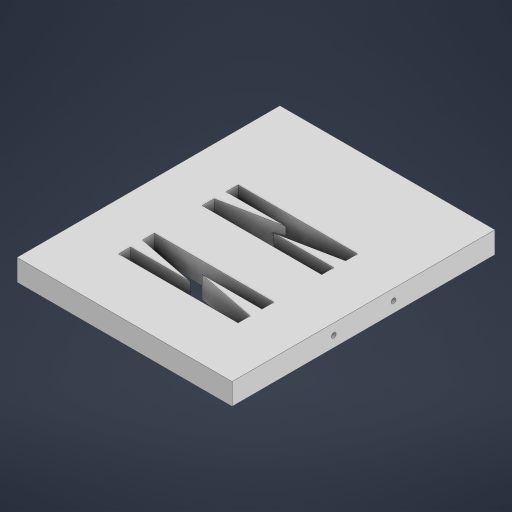
# Autodesk Inventor part: APM_001-3
Saved by Autodesk Inventor 2024 (Build 280153000, 153)
## iProperties
Created: 2023-05-12
Part Number: APM_001-3
Material: Genérico
Document SubType Name: Modeling
Designer: javie
Density: 1 g/cm^3
Appearance: Valor por defecto
Author: javie
Autodesk Inventor part; units mm, degrees
ref_plane "YZ Plane" through (0, 0, 0) normal (1, 0, 0) x (0, 1, 0)
ref_plane "XZ Plane" through (0, 0, 0) normal (0, 1, 0) x (-1, 0, 0)
ref_plane "XY Plane" through (0, 0, 0) normal (0, 0, 1) x (1, 0, 0)
sketch "Boceto1" plane through (0, 0, 0) normal (0, 1, 0) x (-1, 0, 0)
  line L0 (90, 220) -> (-90, 220)
  line L1 (-90, 220) -> (-90, 0)
  line L2 (-90, 0) -> (90, 0)
  line L3 (90, 0) -> (90, 220)
  line L4 (50, 175) -> (-50, 175)
  line L5 (-50, 175) -> (-50, 165)
  line L6 (50, 175) -> (50, 165)
  line L7 (50, 165) -> (0, 165)
  line L8 (50, 155) -> (50, 145)
  line L9 (50, 145) -> (-50, 145)
  line L10 (-50, 145) -> (-50, 155)
  line L11 (-50, 155) -> (0, 155)
  line L12 (0, 155) -> (-50, 165)
  line L13 (0, 165) -> (50, 155)
  line L14 (50, 75) -> (-50, 75)
  line L15 (-50, 75) -> (-50, 85)
  line L16 (50, 75) -> (50, 85)
  line L17 (50, 85) -> (0, 85)
  line L18 (50, 95) -> (50, 105)
  line L19 (50, 105) -> (-50, 105)
  line L20 (-50, 105) -> (-50, 95)
  line L21 (-50, 95) -> (0, 95)
  line L22 (0, 95) -> (-50, 85)
  line L23 (0, 85) -> (50, 95)
  point P0 (0, 0)
  dimension "d0" = 180
  dimension "d1" = 220
  dimension "d2" = 90
  dimension "d3" = 0
  dimension "d5" = 10
  dimension "d6" = 40
  dimension "d7" = 10
  dimension "d8" = 10
  dimension "d9" = 100
  dimension "d11" = 45
  dimension "d13" = 10
  dimension "d14" = 10
  dimension "d15" = 10
  dimension "d16" = 75
  constraints: 48 end point, 6 perpendicular, 2 horizontal, 2 parallel, 2 vertical
  measures "d0" distance of L2.end L1.end
  measures "d1" distance of L1.end L0.end
  measures "d2" distance from line of point (0, 0) L3
  measures "d3" distance from line of L2 point (0, 0)
  measures "d5" distance of L4.end L5.end
  measures "d6" distance between parallel lines of L1 L5
  measures "d7" distance of L4.start L6.end
  measures "d8" distance of L8.start L8.end
  measures "d9" distance of L8.end L9.end
  measures "d11" distance between parallel lines of L0 L4
  measures "d13" distance of L8.start L6.end
  measures "d14" distance of L10.end L5.end
  measures "d15" distance between parallel lines of L9 L11
  measures "d16" distance between parallel lines of L2 L14
extrude "Extrusión1" add sketch "Boceto1" along normal blind 18
sketch "Boceto2" plane through (90, 0, 220) normal (1, 0, 0) x (0, 0, -1)
  line L0 (75, 0) -> (75, 18) projected
  circle A0 centre (135, 9) radius 2
  line L1 (220, 0) -> (220, 18) projected
  circle A1 centre (85, 9) radius 2
  line L2 (0, 0) -> (0, 18) projected
  dimension "d20" = 4
  dimension "d23" = 4
  dimension "d24" = 50
  dimension "d25" = 85
  constraints: 2 centre point
  measures "d20" diameter of A0
  measures "d23" diameter of A1
  measures "d24" distance of A0.centre A1.centre
  measures "d25" distance from line of L2 A1.centre
extrude "Extrusión2" cut sketch "Boceto2" against normal blind 500
